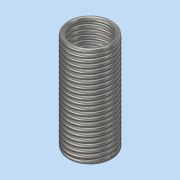
# Autodesk Inventor part: pushSwitchSpring
Saved by Autodesk Inventor 2017 (Build 210142000, 142)
## iProperties
Created: 2016-12-03
Part Number: pushSwitchSpring
Material: Steel, Mild
Document SubType Name: Modeling
Designer: techn
Density: 7.85 g/cm^3
Appearance: Semi-Polished
Author: techn
Autodesk Inventor part; units mm, degrees
ref_plane "YZ Plane" through (0, 0, 0) normal (1, 0, 0) x (0, 1, 0)
ref_plane "XZ Plane" through (0, 0, 0) normal (0, 1, 0) x (-1, 0, 0)
ref_plane "XY Plane" through (0, 0, 0) normal (0, 0, 1) x (1, 0, 0)
sketch "Sketch1" plane through (0, 0, 0) normal (0, 0, 1) x (1, 0, 0)
  circle A0 centre (1.9748, 0) radius 0.2159
  line L0 (0, 0) -> (1.9748, 0)
  line L1 (0, 0) -> (0, 9.525)
  dimension "d0" = 0.4318
  dimension "d1" = 1.9748
  dimension "d2" = 9.525
  constraints: 4 end point, 1 centre point, 1 horizontal, 1 vertical
  measures "d0" diameter of A0
  measures "d1" distance of L0.start L0.end
  measures "d2" distance of L0.start L1.end
coil "Coil1" sketch "Sketch1" operation add axis through (0, 0, 0) along (0, 1, 0) pitch 0.4572 turns 20.833333 hand right
revolve "Revolution1" add sketch "Sketch1" angle 360 about axis through (0, 0, 0) along (0, 1, 0)
sketch "Sketch2" plane through (0.9874, 9.525, 1.7103) normal (0.8660254, 0, -0.5) x (-0.5, 0, -0.8660254)
  circle A0 centre (0, 0) radius 0.2159 projected
  line L0 (0, 0) -> (1.9748, 0)
  line L1 (0, 0) -> (1.9748, 0) construction
  line L2 (1.9748, 0) -> (1.9748, 1.2547)
  point P0 (1.9748, -9.525)
  point P1 (-0.2159, 0)
  dimension "d12" = 1.9748
  dimension "d13" = 0
  constraints: 6 end point, 2 horizontal, 1 collinear, 1 horizontal alignment, 1 perpendicular
  measures "d12" distance of L0.start L0.end
  measures "d13" distance between parallel lines of L0 L1
revolve "Revolution2" add sketch "Sketch2" angle 360 about axis through (0, 9.525, 0) along (0, 1, 0)
body "Solid1"
